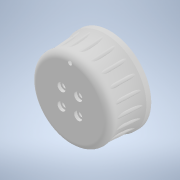
# Autodesk Inventor part: Griff
Saved by Autodesk Inventor 2021 (Build 250183000, 183)
## iProperties
Created: 2024-03-24
Part Number: Griff
Material: Generic
Document SubType Name: Modeling
Designer: Lukas
Density: 1 g/cm^3
Appearance: Default
Author: Lukas
Autodesk Inventor part; units mm, degrees
ref_plane "YZ Plane" through (0, 0, 0) normal (1, 0, 0) x (0, 1, 0)
sketch "Sketch3" plane through (0, 0, 0) normal (0, 1, 0) x (-1, 0, 0)
  line L0 (0, 0) -> (14, 0)
  line L1 (14, 0) -> (17.5, -2)
  line L2 (21, -18) -> (21, -15.5)
  arc A0 (19.8798, -1.3408) -> (21, -15.5) centre (39.0783, -6.9458) ccw
  line L3 (17, 2.5) -> (0, 2.5)
  line L4 (0, 2.5) -> (0, 0)
  line L5 (21, -18) -> (19, -18)
  line L6 (19, -18) -> (19, -16)
  line L7 (19, -16) -> (17.5, -11)
  line L8 (17.5, -11) -> (17.5, -2)
  arc A1 (19.8798, -1.3408) -> (17, 2.5) centre (17, -0.5) ccw
  dimension "d13" = 14
  dimension "d15" = 2.5
  dimension "d21" = 2.5
  dimension "d24" = 17
  dimension "d38" = 20
  dimension "d39" = 18
  dimension "d40" = 17.5
  dimension "d41" = 1.5
  dimension "d42" = 5
  dimension "d43" = 2
  dimension "d44" = 2
  dimension "d58" = 2
  dimension "d59" = 3
  constraints: 18 end point, 4 point on circle, 2 centre point, 2 horizontal, 2 perpendicular, 2 tangent, 2 vertical
  measures "d13" distance of L0.start L0.end
  measures "d15" distance of L2.start L2.end
  measures "d21" distance of L3.end L0.start
  measures "d24" distance of L3.start L3.end
  measures "d38" radius of A0
  measures "d39" distance between parallel lines of L0 L5
  measures "d40" distance between parallel lines of L4 L8
  measures "d41" horizontal distance of L6.end L7.end
  measures "d42" vertical distance of L6.end L7.end
  measures "d43" distance of L5.end L6.end
  measures "d44" distance of L2.start L5.end
  measures "d58" vertical distance of L0.end L1.end
  measures "d59" radius of A1
revolve "Revolution1" add sketch "Sketch3" angle 360 about axis through (0, 0, 2.5) along (0, 0, -1)
sketch "Sketch4" plane through (0, 0, 2.5) normal (0, 0, 1) x (1, 0, 0)
  circle A0 centre (-4.25, 4.25) radius 1.15
  circle A1 centre (-4.25, -4.25) radius 1.15
  circle A2 centre (4.25, -4.25) radius 1.15
  circle A3 centre (4.25, 4.25) radius 1.15
  circle A4 centre (-4.25, 4.25) radius 2.1
  circle A5 centre (4.25, 4.25) radius 2.1
  circle A6 centre (4.25, -4.25) radius 2.1
  circle A7 centre (-4.25, -4.25) radius 2.1
  circle A8 centre (0, 17) radius 1
  point P0 (0, 0)
  dimension "d27" = 8.5
  dimension "d28" = 4.25
  dimension "d29" = 4.25
  dimension "d30" = 8.5
  dimension "d31" = 2.3
  dimension "d32" = 4.2
  dimension "d60" = 17
  dimension "d61" = 2
  constraints: 9 centre point, 6 equal radius, 4 coincident, 3 vertical alignment, 2 horizontal alignment
  measures "d27" distance of A3.centre A0.centre
  measures "d28" horizontal distance of point (0, 0) A0.centre
  measures "d29" horizontal distance of A3.centre point (0, 0)
  measures "d30" distance of A2.centre A3.centre
  measures "d31" diameter of A0
  measures "d32" diameter of A4
  measures "d60" distance of point (0, 0) A8.centre
  measures "d61" diameter of A8
extrude "Extrusion3" cut sketch "Sketch4" against normal through all contours A0 | A1 | A2 | A3
extrude "Extrusion4" cut sketch "Sketch4" against normal blind 1.5
ref_plane "Work Plane2" through (0, 0, -2) normal (0, 0, -1) x (-1, 0, 0)
ref_plane "Work Plane3" through (0, 0, -16) normal (0, 0, -1) x (-1, 0, 0)
sketch "Sketch5" plane through (0, 0, -2) normal (0, 0, -1) x (-1, 0, 0)
  arc A0 (-18.75, 0.9) -> (-18.75, -0.9) centre (-18.75, 0) ccw
  line L0 (-18.75, -0.9) -> (-18.75, 0.9)
  circle A1 centre (0, 0) radius 17.5 projected
  circle A2 centre (0, 0) radius 14 projected
  dimension "d46" = 18.75
  dimension "d47" = 0.9
  constraints: 2 end point, 2 point on circle, 2 vertical alignment, 1 centre point, 1 horizontal alignment, 1 vertical
  measures "d46" distance of point (0, 0) A0.centre
  measures "d47" radius of A0
sketch "Sketch6" plane through (0, 0, -16) normal (0, 0, -1) x (-1, 0, 0)
  line L0 (-19.75, -0.8) -> (-19.75, 0.8)
  arc A0 (-19.75, 0.8) -> (-19.75, -0.8) centre (-19.75, 0) ccw
  circle A1 centre (0, 0) radius 19 projected
  dimension "d48" = 19.75
  dimension "d49" = 0.8
  constraints: 2 end point, 2 point on circle, 1 centre point, 1 coincident, 1 horizontal alignment, 1 midpoint, 1 vertical
  measures "d48" distance from line of point (0, 0) L0
  measures "d49" radius of A0
loft "Loft1" add profiles "Sketch6", "Sketch5" contours A0 L0 / L0 A0
pattern_circular "Circular Pattern1" count 20 over 360 about axis through (0, 0, -10) along (0, 0, 1) of "Loft1"
equation "\"d28\" = 0.5 * d27"
equation "\"d29\" = d28"
equation "\"d30\" = d27"
body "Solid2"
